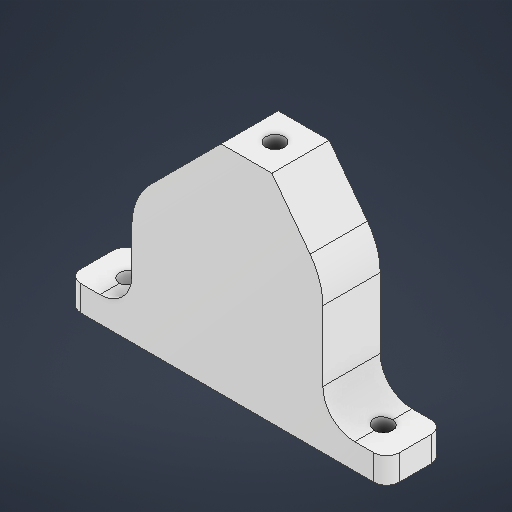
# Autodesk Inventor part: LeftLevelBlock
Saved by Autodesk Inventor 2026.2 (Build 302298000, 298)
## iProperties
Created: 2026-06-02
Part Number: LeftLevelBlock
Material: ABS Plastic
Document SubType Name: Modeling
Designer: gaoet
Density: 1.06 g/cm^3
Appearance: Smooth - White
Author: gaoet
Autodesk Inventor part; units mm, degrees
ref_plane "YZ Plane" through (0, 0, 0) normal (1, 0, 0) x (0, 1, 0)
ref_plane "XZ Plane" through (0, 0, 0) normal (0, 1, 0) x (-1, 0, 0)
ref_plane "XY Plane" through (0, 0, 0) normal (0, 0, 1) x (1, 0, 0)
sketch "Sketch1" plane through (0, 0, 0) normal (0, 0, 1) x (1, 0, 0)
  line L0 (-25, -5) -> (25, -5)
  line L1 (25, -5) -> (25, 5)
  line L2 (25, 5) -> (-25, 5)
  line L3 (-25, 5) -> (-25, -5)
  line L4 (-25, -5) -> (25, 5) construction
  line L5 (25, -5) -> (-25, 5) construction
  line L6 (-25, 5) -> (-1, 29)
  line L7 (-1, 29) -> (7, 29)
  line L8 (7, 29) -> (25, 5)
  line L9 (3, 29) -> (3, 5) construction
  point P0 (0, 0)
  dimension "d0" = 28
  dimension "d1" = 50
  dimension "d2" = 34
  dimension "d3" = 8
  dimension "d4" = 10
  constraints: 20 end point, 3 midpoint, 2 horizontal, 2 parallel, 2 perpendicular, 1 point on line
  measures "d0" distance between parallel lines of L3 L9
  measures "d1" distance of L0.start L0.end
  measures "d2" distance between parallel lines of L0 L7
  measures "d3" distance of L6.end L7.end
  measures "d4" distance of L0.end L1.end
extrude "Extrusion1" add sketch "Sketch1" along normal blind 9
sketch "Sketch2" plane through (-25, -5, 0) normal (0, -1, 0) x (1, 0, 0)
  line L0 (0, 0) -> (50, 0) projected
  line L1 (50, 0) -> (50, 9) projected
  line L2 (0, 9) -> (50, 9) projected
  line L3 (0, 0) -> (0, 9) projected
  point P0 (25, 0)
  point P1 (5, 4.5)
  point P2 (25, 4.5)
  point P3 (45, 4.5)
  point P4 (50, 4.5)
  dimension "d7" = 20
  dimension "d8" = 20
  dimension "d9" = 5
  constraints: 3 horizontal alignment, 1 midpoint
  measures "d7" distance of point (45, 4.5) point (25, 4.5)
  measures "d8" distance of point (5, 4.5) point (25, 4.5)
  measures "d9" distance from line of L1 point (45, 4.5)
hole "Hole1" at (20, -5, 4.5) at (-20, -5, 4.5) at (0, -5, 4.5) direction (0, 1, 0) diameter 2.9 depth 10
sketch "Sketch3" plane through (-1, 29, 0) normal (0, 1, 0) x (1, 0, 0)
  line L0 (8, 0) -> (0, 0) projected
  line L1 (0, 0) -> (0, -9) projected
  line L2 (8, -9) -> (0, -9) projected
  line L3 (8, 0) -> (8, -9) projected
  point P0 (1, 0)
  point P1 (4, -4.5)
  point P2 (8, -4.5)
  point P3 (4, 0)
  constraints: 2 midpoint, 1 horizontal alignment, 1 vertical alignment
hole "Hole2" at (3, 29, 4.5) direction (0, -1, 0) diameter 2.9 depth 20
sketch "Sketch4" plane through (0, 0, 0) normal (0, 0, -1) x (-1, 0, 0)
  line L0 (-18.55, -5) -> (-21.45, -5) projected
  line L1 (-21.45, 5) -> (-18.55, 5) projected
  line L2 (-25, -5) -> (-25, 5) projected
  line L3 (-25, -1) -> (-15, -1)
  line L4 (-15, -1) -> (-15, 18.3333)
  line L5 (25, -5) -> (-25, -5) projected
  line L6 (-7, 29) -> (1, 29) projected
  line L7 (-25, 5) -> (-7, 29) projected
  line L8 (-25, -5) -> (-25, 5) projected
  line L9 (25, -5) -> (-25, -5) projected
  line L10 (25, 5) -> (25, -5) projected
  line L11 (1, 29) -> (25, 5) projected
  line L12 (21.45, 5) -> (21.45, -5) projected
  line L13 (18.55, 5) -> (18.55, -5) projected
  line L14 (-15, -1) -> (25, -1)
  line L15 (15, -1) -> (15, 15)
  point P0 (0, 0)
  dimension "d25" = 3.55
  dimension "d26" = 4
  dimension "d27" = 3.55
  constraints: 8 end point, 5 point on line, 3 perpendicular, 1 vertical
  measures "d25" distance from line of L4 L1.end
  measures "d26" distance between parallel lines of L5 L3
  measures "d27" distance between parallel lines of L13 L15
extrude "Extrusion2" cut sketch "Sketch4" against normal through all contours L14 L15 L11 L10 | L2 L7 L4 L3
fillet "Fillet2" radius 5 2 edges at (15, -1, 4.5) (-15, -1, 4.5)
fillet "Fillet3" radius 2 4 edges at (25, -3, 0) (25, -3, 9) (-25, -3, 0) (-25, -3, 9)
fillet "Fillet4" radius 10 2 edges at (-15, 15, 4.5) (15, 18.3333, 4.5)
equation "\"d8\" = d7"
equation "\"d27\" = d25"
body "Solid1"
